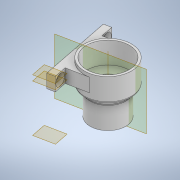
# Autodesk Inventor part: CFT_koppelstuk
Saved by Autodesk Inventor 2020.5 (Build 245400000, 400)
## iProperties
Created: 2022-03-03
Part Number: CFT_koppelstuk
Material: Generic
Document SubType Name: Modeling
Designer: EDDY
Density: 1 g/cm^3
Appearance: Default
Author: EDDY
## iProperties of the stored document _3DPrint.ipt
Created: 2022-03-03
Part Number: _3DPrint
Material: Generic
Document SubType Name: Modeling
Designer: EDDY
Density: 1 g/cm^3
Appearance: Default
Author: EDDY
Autodesk Inventor part; units mm, degrees
ref_plane "YZ Plane" through (0, 0, 0) normal (1, 0, 0) x (0, 1, 0)
ref_plane "XZ Plane" through (0, 0, 0) normal (0, 1, 0) x (-1, 0, 0)
ref_plane "XY Plane" through (0, 0, 0) normal (0, 0, 1) x (1, 0, 0)
sketch "Sketch1" plane through (0, 0, 0) normal (0, 0, 1) x (1, 0, 0)
  line L0 (0, 0) -> (0, 56.35)
  line L1 (0, 56.35) -> (26.1, 56.35)
  line L2 (26.1, 56.35) -> (26.1, 31.35)
  line L3 (26.1, 31.35) -> (19.75, 25)
  line L4 (19.75, 25) -> (19.75, 0)
  line L5 (19.75, 0) -> (0, 0)
  dimension "d1" = 39.5
  dimension "d3" = 45
  dimension "d5" = 52.2
  dimension "d6" = 25
  constraints: 12 end point, 2 perpendicular, 1 horizontal, 1 parallel, 1 vertical
  measures "d1" diameter of L4 L0
  measures "d3" angle of L0 L3
  measures "d5" diameter of L2 L0
  measures "d6" distance of L1.end L2.end
revolve "Revolution1" add sketch "Sketch1" angle 360 about axis through (0, 0, 0) along (0, -1, 0)
fillet "Fillet2" radius 2 1 edges at (-19.75, 25, 0)
fillet "Fillet3" radius 2 1 edges at (-26.1, 31.35, 0)
shell "Shell2" thickness 2.5 removed faces 2 at (7.4507, 56.35, 1.961) at (5.8293, 0, 3.0594)
ref_plane "Work Plane4" through (-19.7215, 58.7231, 59.4617) normal (0, 1, 0) x (-0.9806, 0, 0.1963)
ref_plane "Work Plane2" through (-19.7215, 0.4561, 59.4617) normal (0, 1, 0) x (-0.9806, 0, 0.1963)
ref_plane "Work Plane5" through (-19.7215, 52.7231, 59.4617) normal (0, 1, 0) x (-0.9806, 0, 0.1963)
sketch "Sketch5" plane through (-19.7215, 52.7231, 59.4617) normal (0, 1, 0) x (-0.9806, 0, 0.1963)
  circle A0 centre (-31.0082, -54.4346) radius 26.1 projected
  line L0 (-8, -28.3346) -> (-8, -14.4346)
  line L1 (-8, -14.4346) -> (0, -14.4346)
  line L2 (0, -14.4346) -> (0, -94.4346)
  line L3 (0, -94.4346) -> (-8, -94.4346)
  line L4 (0, 0) -> (0, -15) projected
  line L5 (-8, -94.4346) -> (-8, -80.5346)
  line L6 (-8, -80.5346) -> (-31.0082, -80.5346)
  line L7 (-31.0082, -28.3346) -> (-8, -28.3346)
  point P0 (-31.0082, -54.4346)
  dimension "d20" = 40
  dimension "d21" = 40
  dimension "d22" = 8
  constraints: 14 end point, 3 perpendicular, 2 collinear, 2 horizontal, 2 point on circle, 2 vertical
  measures "d20" distance from line of L1 point (-31.008, -54.435)
  measures "d21" distance from line of L3 point (-31.008, -54.435)
  measures "d22" distance of L2.end L3.end
extrude "Extrusion2" add sketch "Sketch5" against normal blind 15 contours A0 L7 L0 L1 L2 L3 L5 L6
sketch "Sketch6" plane through (-27.6833, 37.7231, -21.0766) normal (0.9806, 0, -0.1963) x (-0.1963, 0, -0.9806)
  point P0 (-26.1, -37.7231)
ref_plane "Work Plane6" through (0, 43.85, 0) normal (-0.1963, 0, -0.9806) x (0, -1, 0)
sketch "Sketch7" plane through (-27.6833, 37.7231, -21.0766) normal (0.9806, 0, -0.1963) x (-0.1963, 0, -0.9806)
  line L0 (0, 15) -> (13.9, 15) projected
  line L1 (13.9, 15) -> (13.9, 0) projected
  point P0 (-26.1, -37.7231)
  point P1 (6.9, 7.5)
  dimension "d27" = 7.5
  dimension "d35" = 7
  measures "d27" distance from line of L0 point (6.9, 7.5)
  measures "d35" distance from line of L1 point (6.9, 7.5)
hole "Hole1" at (-29.0375, 45.2231, -27.8424) direction (-0.9806, 0, 0.1963) diameter 4.5 end through all
mirror "Mirror1" about plane through (0, 43.85, 0) normal (-0.1963, 0, -0.9806) of "Hole1"
chamfer "Chamfer2" distance 4 angle 45 2 edges at (-28.5959, 45.2231, -25.6362) (-16.5256, 45.2231, 34.6677)
body "Solid1"
